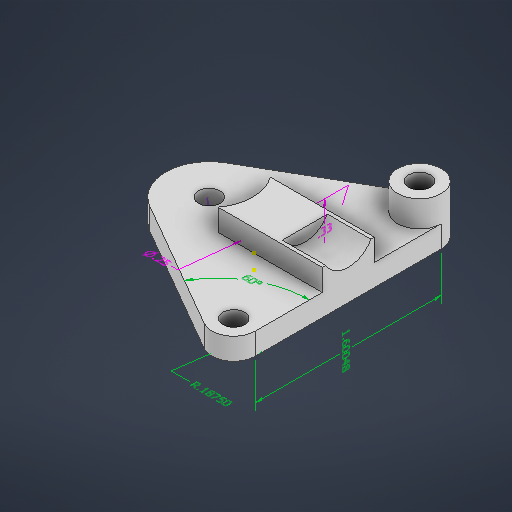
# Autodesk Inventor part: EndTop3
Saved by Autodesk Inventor 2026 (Build 300175000, 175)
## iProperties
Created: 2025-04-09
Part Number: EndTop3
Material: Generic
Document SubType Name: Modeling
Designer: jjgen
Density: 1 g/cm^3
Appearance: Default
Author: jjgen
Autodesk Inventor part; units mm, degrees
ref_plane "YZ Plane" through (0, 0, 0) normal (1, 0, 0) x (0, 1, 0)
ref_plane "XZ Plane" through (0, 0, 0) normal (0, 1, 0) x (-1, 0, 0)
ref_plane "XY Plane" through (0, 0, 0) normal (0, 0, 1) x (1, 0, 0)
sketch "Sketch1" plane through (0, 0, 0) normal (0, 1, 0) x (-1, 0, 0)
  line L0 (0, -5.4993) -> (0, -32.6007)
  line L1 (4.7625, -35.3504) -> (23.4706, -24.5493)
  line L2 (0, -38.1) -> (21.6022, -38.1) construction
  line L3 (23.4706, -13.5507) -> (4.7625, -2.7496)
  arc A0 (4.7625, -2.7496) -> (0, -5.4993) centre (3.175, -5.4993) ccw
  arc A1 (0, -32.6007) -> (4.7625, -35.3504) centre (3.175, -32.6007) ccw
  arc A2 (23.4706, -24.5493) -> (23.4706, -13.5507) centre (20.2956, -19.05) ccw
  line L4 (1.5875, -35.3504) -> (4.8895, -35.3504) construction
  line L5 (26.6456, -19.05) -> (20.2956, -19.05)
  circle A3 centre (20.2956, -19.05) radius 6.35
  circle A4 centre (20.2956, -19.05) radius 1.5875
  circle A5 centre (3.175, -5.4993) radius 3.175
  circle A6 centre (3.175, -5.4993) radius 1.5875
  circle A7 centre (3.175, -32.6007) radius 3.175
  circle A8 centre (3.175, -32.6007) radius 1.5875
  point P0 (0, 0)
  point P1 (32.9956, -19.05)
  point P2 (0, -32.6007)
  point P3 (4.7625, -2.7496)
  point P4 (4.7625, -2.7496)
  point P5 (0, -32.6007)
  dimension "d9" = 38.1
  dimension "d10" = 38.1
  dimension "d11" = 30
  dimension "d12" = 3.175
  dimension "d13" = 6.35
  dimension "d21" = 3.175
  dimension "d22" = 3.175
  dimension "d23" = 3.175
  constraints: 12 end point, 8 centre point, 8 point on circle, 6 coincident, 6 point on line, 6 tangent, 3 horizontal, 2 equal radius, 1 equal length, 1 vertical, 3 other
  measures "d9" distance of point (0, 0) L2.start
  measures "d10" distance of L2.start point (32.996, -19.05)
  measures "d11" angle of L2 L1
  measures "d12" radius of A0
  measures "d13" radius of A2
  measures "d21" diameter of A4
  measures "d22" diameter of A6
  measures "d23" diameter of A8
extrude "Extrusion1" add sketch "Sketch1" along normal blind 6.35 contours A0 A5 | A7 A1 | A2 A3
extrude "Extrusion2" add sketch "Sketch1" along normal blind 3.175 contours A5 L3 A3 L1 A7 L0
sketch "Sketch2" plane through (0, 3.175, 0) normal (0, 1, 0) x (1, 0, 0)
  arc A0 (-23.4706, 13.5507) -> (-23.4706, 24.5493) centre (-20.2956, 19.05) ccw projected
  line L0 (-13.9456, 19.05) -> (0, 19.05)
  line L1 (0, 5.4993) -> (0, 32.6007) projected
  line L2 (-20.2956, 19.05) -> (-20.2956, 25.4)
  line L3 (0, 19.05) -> (0, 24.765)
  line L4 (0, 19.05) -> (0, 13.335)
  line L5 (-13.9456, 19.05) -> (-13.9456, 13.335)
  line L6 (-13.9456, 19.05) -> (-13.9456, 24.765)
  line L7 (-13.9456, 19.05) -> (-10.1478, 19.05)
  line L8 (-10.1478, 13.335) -> (-10.1478, 24.765)
  line L9 (0, 13.335) -> (-17.5277, 13.335)
  line L10 (0, 24.765) -> (-17.5277, 24.765)
  point P0 (0, 0)
  dimension "d28" = 5.715
  dimension "d29" = 5.715
  constraints: 20 end point, 7 point on line, 4 point on circle, 1 horizontal, 1 midpoint, 1 parallel, 1 tangent, 1 vertical
  measures "d28" distance of L0.end L3.end
  measures "d29" distance of L0.end L4.end
extrude "Extrusion3" add sketch "Sketch2" along normal blind 6.35 contours A0 L5 L9 | L6 L10 L8 L0 | L0 L8 L9 L5 | A0 L10 L6
sketch "Sketch3" plane through (0, 3.175, 0) normal (0, 1, 0) x (1, 0, 0)
  line L0 (-10.1478, 13.335) -> (0, 13.335)
  line L1 (0, 5.4993) -> (0, 32.6007) projected
  line L2 (-10.1478, 24.765) -> (-10.1478, 13.335) projected
  line L3 (-10.1478, 24.765) -> (0, 24.765)
  line L4 (0, 24.765) -> (0, 13.335)
  point P0 (0, 0)
  constraints: 6 end point, 2 horizontal, 1 perpendicular, 1 point on line
extrude "Extrusion4" add sketch "Sketch3" along normal blind 6.35
sketch "Sketch4" plane through (0, 0, -5.4993) normal (1, 0, 0) x (0, 0, -1)
  line L0 (7.8357, 9.525) -> (19.2657, 9.525) projected
  line L1 (13.5507, 9.525) -> (13.5507, 12.065)
  circle A0 centre (13.5507, 12.065) radius 5.715
  point P0 (-5.4993, 0)
  point P1 (8.4312, 9.525)
  point P2 (18.6703, 9.525)
  dimension "d34" = 2.54
  constraints: 2 end point, 1 centre point, 1 coincident, 1 midpoint, 1 vertical
  measures "d34" distance of L1.start L1.end
extrude "Extrusion5" cut sketch "Sketch4" against normal blind 10.16 contours L0 A0 picked at (16.7053, 9.1339)
sketch "Sketch5" plane through (0, 9.525, 0) normal (0, 1, 0) x (1, 0, 0)
  point P0 (0, 0)
sketch "Sketch6" plane through (0, 9.525, 0) normal (0, 1, 0) x (1, 0, 0)
  arc A0 (-17.5277, 13.335) -> (-17.5277, 24.765) centre (-20.2956, 19.05) ccw projected
  line L0 (-17.5277, 13.335) -> (0, 13.335) projected
  line L1 (-17.5277, 13.335) -> (0, 13.335)
  line L2 (-17.5277, 24.765) -> (0, 24.765) projected
  line L3 (0, 13.335) -> (0, 24.765)
  line L4 (0, 24.765) -> (-17.5277, 24.765)
  arc A1 (-17.5277, 24.765) -> (-23.4706, 24.5493) centre (-20.2956, 19.05) ccw projected
  arc A2 (-17.5277, 13.335) -> (-17.5277, 24.765) centre (-20.2956, 19.05) ccw
  point P0 (0, 0)
  constraints: 6 end point, 2 collinear, 2 point on circle, 1 centre point, 1 perpendicular
extrude "Extrusion6" cut sketch "Sketch6" against normal blind 6.35
sketch "Sketch7" plane through (0, 3.175, 0) normal (0, 1, 0) x (1, 0, 0)
  line L0 (-13.676, 19.05) -> (0, 19.05)
  line L1 (0, 5.4993) -> (0, 32.6007) projected
  line L2 (0, 19.05) -> (0, 22.8639)
  line L3 (0, 22.8639) -> (-15.2185, 22.8639)
  arc A0 (-23.4706, 13.5507) -> (-23.4706, 24.5493) centre (-20.2956, 19.05) ccw projected
  line L4 (0, 19.05) -> (0, 15.24)
  line L5 (0, 15.24) -> (-15.2185, 15.24)
  point P0 (0, 0)
  point P1 (-15.2156, 15.24)
  dimension "d39" = 3.81
  constraints: 10 end point, 2 perpendicular, 1 midpoint, 1 point on circle, 1 point on line, 1 vertical
  measures "d39" distance of L0.end L4.end
extrude "Extrusion7" add sketch "Sketch7" along normal blind 6.35
sketch "Sketch8" plane through (0, 0, -5.4993) normal (1, 0, 0) x (0, 0, -1)
  line L0 (9.7407, 9.525) -> (17.3646, 9.525) projected
  circle A0 centre (13.5527, 9.525) radius 2.9247
  point P0 (-5.4993, 0)
  point P1 (16.4774, 9.525)
  point P2 (10.628, 9.525)
  constraints: 1 centre point, 1 midpoint
extrude "Extrusion8" cut sketch "Sketch8" against normal blind 6.35 contours L0 A0 picked at (12.9156, 8.0363)
sketch "Sketch9" plane through (-3.175, 6.35, -5.4993) normal (0, 1, 0) x (1, 0, 0)
  circle A0 centre (0, 0) radius 1.5875 projected
  circle A1 centre (0, 0) radius 3.1908
  point P0 (3.175, -5.4993)
  constraints: 1 centre point, 1 coincident
extrude "Extrusion9" add sketch "Sketch9" along normal blind 6.35
sketch "Sketch10" plane through (-6.35, 0, -5.4993) normal (1, 0, 0) x (0, 0, -1)
  point P0 (-5.4993, 0)
sketch "Sketch11" plane through (-6.35, 0, -5.4993) normal (1, 0, 0) x (0, 0, -1)
  line L0 (10.628, 9.525) -> (16.4774, 9.525) projected
  circle A0 centre (13.5527, 9.525) radius 2.9247
  point P0 (-5.4993, 0)
  constraints: 1 centre point, 1 midpoint
extrude "Extrusion10" add sketch "Sketch11" along normal blind 6.35 contours L0 A0 picked at (12.9156, 8.0363)
sketch "Sketch12" plane through (0, 0, -5.4993) normal (1, 0, 0) x (0, 0, -1)
  line L0 (9.7407, 9.525) -> (17.3646, 9.525) projected
  line L1 (13.5527, 9.525) -> (13.5527, 11.43)
  circle A0 centre (13.5527, 11.43) radius 2.8589
  circle A1 centre (13.5527, 11.43) radius 3.8119
  point P0 (-5.4993, 0)
  point P1 (11.4209, 9.525)
  point P2 (10.2509, 9.525)
  point P3 (16.8545, 9.525)
  point P4 (15.6845, 9.525)
  dimension "d48" = 1.905
  constraints: 2 centre point, 2 coincident, 2 end point, 1 midpoint, 1 vertical
  measures "d48" distance of L1.start L1.end
extrude "Extrusion11" cut sketch "Sketch12" against normal blind 6.35 contours L0 A0 A1 | A0 L0 | L0 A0 picked at (13.667, 7.9598)
sketch "Sketch13" plane through (-3.175, 12.7, -5.4993) normal (0, 1, 0) x (1, 0, 0)
  point P0 (3.175, -5.4993)
sketch "Sketch14" plane through (-3.175, 12.7, -5.4993) normal (0, 1, 0) x (1, 0, 0)
  point P0 (3.175, -5.4993)
sketch "Sketch15" plane through (0, 9.525, 0) normal (0, 1, 0) x (1, 0, 0)
  line L0 (-32.2376, -8.2209) -> (5.0804, -8.2209)
  line L1 (5.0804, -8.2209) -> (5.0804, 48.4404)
  line L2 (5.0804, 48.4404) -> (-32.2376, 48.4404)
  line L3 (-32.2376, 48.4404) -> (-32.2376, -8.2209)
  point P0 (0, 0)
  constraints: 8 end point, 2 parallel, 1 horizontal, 1 perpendicular
extrude "Extrusion12" cut sketch "Sketch15" against normal blind 6.35
sketch "Sketch16" plane through (-3.175, 12.7, -5.4993) normal (0, 1, 0) x (1, 0, 0)
  line L0 (-6.5879, -11.43) -> (8.5583, -11.43)
  line L1 (8.5583, -11.43) -> (8.5583, 13.0229)
  line L2 (8.5583, 13.0229) -> (-6.5879, 13.0229)
  line L3 (-6.5879, 13.0229) -> (-6.5879, -11.43)
  point P0 (3.175, -5.4993)
  constraints: 8 end point, 2 parallel, 1 horizontal, 1 perpendicular
extrude "Extrusion13" cut sketch "Sketch16" against normal blind 6.35
sketch "Sketch17" plane through (0, 3.175, 0) normal (0, 1, 0) x (1, 0, 0)
  circle A0 centre (-3.175, 32.6007) radius 1.5875 projected
  circle A1 centre (-3.175, 32.6007) radius 3.175
  circle A2 centre (-3.175, 32.6007) radius 1.5875
  point P0 (0, 0)
  dimension "d67" = 3.175
  constraints: 2 centre point, 2 coincident
  measures "d67" diameter of A2
extrude "Extrusion14" add sketch "Sketch17" along normal blind 3.81
sketch "Sketch18" plane through (0, 3.175, 0) normal (0, 1, 0) x (1, 0, 0)
  circle A0 centre (-20.2956, 19.05) radius 1.5875 projected
  line L0 (-20.2956, 19.05) -> (-13.9456, 19.05)
  line L1 (-13.9456, 19.05) -> (0, 19.05)
  line L2 (0, 5.4993) -> (0, 32.6007) projected
  line L3 (-13.9456, 19.05) -> (-13.9456, 22.86)
  line L4 (-13.9456, 22.86) -> (0, 22.86)
  line L5 (-13.9456, 19.05) -> (-13.9456, 15.24)
  line L6 (-13.9456, 15.24) -> (0, 15.24)
  line L7 (0, 15.24) -> (0, 22.86)
  point P0 (0, 0)
  dimension "d70" = 6.35
  dimension "d71" = 3.81
  dimension "d72" = 3.81
  constraints: 14 end point, 4 perpendicular, 2 point on line, 1 horizontal, 1 midpoint
  measures "d70" distance of L0.start L0.end
  measures "d71" distance of L0.end L3.end
  measures "d72" distance of L0.end L5.end
extrude "Extrusion15" add sketch "Sketch18" along normal blind 3.175 contours L3 L4 L2 L1 | L1 L2 L6 L5
sketch "Sketch19" plane through (0, 0, -5.4993) normal (1, 0, 0) x (0, 0, -1)
  line L0 (9.7407, 6.35) -> (17.3607, 6.35) projected
  line L1 (13.5507, 6.35) -> (13.5507, 8.255)
  circle A0 centre (13.5507, 8.255) radius 3.81
  point P0 (-5.4993, 0)
  point P1 (10.2512, 6.35)
  point P2 (16.8503, 6.35)
  dimension "d75" = 1.905
  dimension "d76" = 7.62
  constraints: 2 end point, 1 centre point, 1 coincident, 1 midpoint, 1 vertical
  measures "d75" distance of L1.start L1.end
  measures "d76" diameter of A0
extrude "Extrusion16" cut sketch "Sketch19" against normal blind 6.35 contours L0 A0 picked at (11.5271, 6.1135)
sketch "Sketch20" plane through (0, 3.175, 0) normal (0, 1, 0) x (1, 0, 0)
  arc A0 (-23.4706, 24.5493) -> (-23.4706, 13.5507) centre (-20.2956, 19.05) ccw projected
  line L0 (-26.6456, 19.05) -> (-20.2956, 19.05)
  circle A1 centre (-20.2956, 19.05) radius 1.5875 projected
  circle A2 centre (-20.2956, 19.05) radius 6.35
  line L1 (-13.9456, 22.86) -> (0, 22.86) projected
  line L2 (-13.9456, 22.86) -> (-15.2156, 22.86)
  line L3 (-13.9456, 15.24) -> (-15.2156, 15.24)
  arc A3 (-15.2156, 15.24) -> (-15.2156, 22.86) centre (-20.2956, 19.05) ccw
  arc A4 (-15.2156, 15.24) -> (-15.2156, 22.86) centre (-20.2956, 19.05) ccw
  point P0 (0, 0)
  constraints: 7 point on circle, 6 end point, 3 centre point, 2 horizontal, 1 coincident, 1 collinear, 1 concentric
sketch "Sketch21" plane through (0, 3.175, 0) normal (0, 1, 0) x (1, 0, 0)
  line L0 (-13.9456, 15.24) -> (-15.2035, 15.24)
  line L1 (-13.9456, 15.24) -> (-15.2035, 15.24)
  line L2 (-13.9456, 15.24) -> (-13.9456, 22.86) projected
  line L3 (-13.9456, 22.86) -> (-15.2035, 22.86)
  line L4 (-15.2035, 22.86) -> (-15.2035, 15.24)
  line L5 (-15.2035, 15.24) -> (-13.9456, 15.24)
  line L6 (-13.9456, 15.24) -> (-13.9456, 22.86)
  line L7 (-13.9456, 22.86) -> (-15.2035, 22.86)
  line L8 (-15.2035, 22.86) -> (-15.2035, 15.24)
  point P0 (0, 0)
  constraints: 16 end point, 4 equal length, 3 horizontal, 1 perpendicular
extrude "Extrusion17" add sketch "Sketch21" along normal blind 3.175
sketch "Sketch22" plane through (0, 6.35, 0) normal (0, 1, 0) x (1, 0, 0)
  arc A0 (-23.4706, 24.5493) -> (-23.4706, 13.5507) centre (-20.2956, 19.05) ccw projected
  line L0 (-26.6456, 19.05) -> (-20.2956, 19.05)
  circle A1 centre (-20.2956, 19.05) radius 1.5875 projected
  circle A2 centre (-20.2956, 19.05) radius 6.35
  point P0 (0, 0)
  constraints: 2 end point, 1 centre point, 1 coincident, 1 horizontal, 1 point on circle
extrude "Extrusion18" cut sketch "Sketch22" against normal blind 3.175
scale "Scale1" factors (1.5, 1.5, 1.5) then translate (7.0583, 0, 14.9749) bodies 1
body "Solid1"
